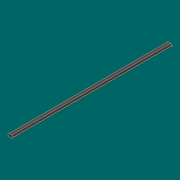
# Autodesk Inventor part: topBottomORing
Saved by Autodesk Inventor 2016 (Build 200138000, 138)
## iProperties
Created: 2015-10-19
Part Number: topBottomORing
Material: Rubber
Document SubType Name: Modeling
Designer: Sawaiz
Density: 0.93 g/cm^3
Appearance: Rubber - Black
Author: Sawaiz
Autodesk Inventor part; units mm, degrees
ref_plane "YZ Plane" through (0, 0, 0) normal (1, 0, 0) x (0, 1, 0)
ref_plane "XZ Plane" through (0, 0, 0) normal (0, 1, 0) x (-1, 0, 0)
ref_plane "XY Plane" through (0, 0, 0) normal (0, 0, 1) x (1, 0, 0)
sketch "Sketch1" plane through (0, 0, 0) normal (0, 0, 1) x (1, 0, 0)
  line L0 (49.8475, -1.5875) -> (-49.8475, -1.5875)
  line L1 (-49.8475, -1.5875) -> (-49.8475, 1.5875)
  line L2 (-49.8475, 1.5875) -> (49.8475, 1.5875)
  line L3 (49.8475, 1.5875) -> (49.8475, -1.5875)
  line L4 (49.8475, -1.5875) -> (-49.8475, 1.5875) construction
  line L5 (-49.8475, -1.5875) -> (49.8475, 1.5875) construction
  point P0 (0, 0)
  dimension "d0" = 99.695
  dimension "d1" = 3.175
  constraints: 12 end point, 2 midpoint, 2 parallel, 1 horizontal, 1 perpendicular
  measures "d0" distance of L1.end L2.end
  measures "d1" distance of L0.end L1.end
extrude "Extrusion1" add sketch "Sketch1" along normal blind 1.905
fillet "Fillet1" radius 0.7937 4 edges at (0, 1.5875, 1.905) (0, -1.5875, 1.905) (0, 1.5875, 0) (0, -1.5875, 0)
equation "\"d1\" = oRingWidth"
equation "\"d4\" = 0.25 * oRingWidth"
equation "\"acrylicThickness\" = 6.35"
equation "\"height\" = 101.6"
equation "\"width\" = 101.6"
equation "\"depth\" = 101.6"
equation "\"mirrorAngle\" = 5deg"
equation "\"detectorWidth\" = 52"
equation "\"detectorHeight\" = 52"
equation "\"mirrorThickness\" = 3"
equation "\"fresnelThickness\" = 0.1"
equation "\"focalLength\" = 76.2"
equation "\"ior\" = 1.49"
equation "\"centerThickness\" = 1.524"
equation "\"fresnelAngle\" = 90deg"
equation "\"fresnelEffectiveDiameter\" = 76.2"
equation "\"mirrorSuppourtWidth\" = 38.1"
equation "\"backGrooveBit\" = 4.8006"
equation "\"sensorHolderWidth\" = 88.9"
equation "\"sensorHolderHeight\" = 88.9"
equation "\"sensorHolderSensorHeight\" = 53.975"
equation "\"sensorHolderSensorWidth\" = 53.975"
equation "\"oRingWidth\" = 3.175"
equation "\"sensorHolderORingID\" = 203.2"
equation "\"sensorHolderFlushORingID\" = 254"
equation "\"frontBackORingID\" = 419.1"
equation "\"mirrorGroove\" = 19.05"
equation "\"backMirrorGroove\" = 6.35"
equation "\"mirrorGrooveFillet\" = 6.35"
equation "\"fresnelChamfer\" = 6.35"
equation "\"mirrorGrooveDrill\" = 6.35"
equation "\"mirrorGrooveMill\" = 3.175"
body "Solid1"
